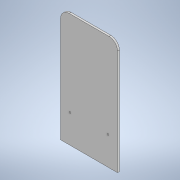
# Autodesk Inventor part: mountPlate
Saved by Autodesk Inventor 2020 (Build 240168000, 168)
## iProperties
Created: 2020-07-21
Part Number: mountPlate
Material: Generic
Document SubType Name: Modeling
Designer: lu0248
Density: 1 g/cm^3
Appearance: Default
Author: lu0248
Autodesk Inventor part; units mm, degrees
ref_plane "YZ Plane" through (0, 0, 0) normal (1, 0, 0) x (0, 1, 0)
ref_plane "XZ Plane" through (0, 0, 0) normal (0, 1, 0) x (-1, 0, 0)
ref_plane "XY Plane" through (0, 0, 0) normal (0, 0, 1) x (1, 0, 0)
sketch "Sketch1" plane through (0, 0, 0) normal (0, 0, 1) x (1, 0, 0)
  line L0 (-150, 0) -> (150, 0)
  line L1 (150, 0) -> (150, 600)
  line L2 (150, 600) -> (-150, 600)
  line L3 (-150, 600) -> (-150, 0)
  point P0 (0, 0)
  dimension "d0" = 600
  dimension "d1" = 300
  dimension "d2" = 150
  constraints: 8 end point, 2 parallel, 1 horizontal, 1 midpoint, 1 perpendicular
  measures "d0" distance of L2.end L0.start
  measures "d1" distance of L1.end L2.end
  measures "d2" distance from line of point (0, 0) L3
extrude "Extrusion1" add sketch "Sketch1" along normal blind 10
fillet "Fillet1" radius 45 2 edges at (150, 600, 5) (-150, 600, 5)
sketch "Sketch2" plane through (0, 0, 10) normal (0, 0, 1) x (1, 0, 0)
  line L0 (-150, 555) -> (-150, 0) projected
  line L1 (150, 0) -> (150, 555) projected
  line L2 (-150, 0) -> (150, 0) projected
  point P0 (0, 0)
  point P1 (-100, 150)
  point P2 (100, 150)
  dimension "d6" = 50
  dimension "d7" = 50
  dimension "d8" = 150
  dimension "d9" = 150
  measures "d6" distance from line of L0 point (-100, 150)
  measures "d7" distance from line of L1 point (100, 150)
  measures "d8" distance from line of L2 point (100, 150)
  measures "d9" distance from line of L2 point (-100, 150)
hole "Hole1" at (-100, 150, 10) at (100, 150, 10) direction (0, 0, -1) diameter 8 depth 60
equation "\"d0\" = partHeight"
equation "\"d1\" = partWidth"
equation "\"d2\" = 0.5 * partWidth"
equation "\"d3\" = thickness"
equation "\"partWidth\" = 300"
equation "\"partHeight\" = 600"
equation "\"thickness\" = 10"
equation "\"holeHeight\" = 1"
equation "\"ribSpacing\" = 1"
equation "\"ribThickness\" = 1"
body "Solid1"
